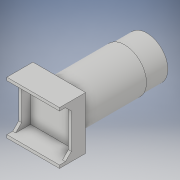
# Autodesk Inventor part: More Accurate Button
Saved by Autodesk Inventor 2018 (Build 220112000, 112)
## iProperties
Created: 2019-09-13
Part Number: More Accurate Button
Material: Generic
Document SubType Name: Modeling
Designer: Jacob
Density: 1 g/cm^3
Appearance: Default
Author: Jacob
Autodesk Inventor part; units mm, degrees
ref_plane "YZ Plane" through (0, 0, 0) normal (1, 0, 0) x (0, 1, 0)
ref_plane "XZ Plane" through (0, 0, 0) normal (0, 1, 0) x (-1, 0, 0)
ref_plane "XY Plane" through (0, 0, 0) normal (0, 0, 1) x (1, 0, 0)
sketch "Sketch1" plane through (0, 0, 0) normal (0, 0, 1) x (1, 0, 0)
  line L0 (-8.875, 8.875) -> (8.875, 8.875)
  line L1 (8.875, 8.875) -> (8.875, -8.875)
  line L2 (8.875, -8.875) -> (-8.875, -8.875)
  line L3 (-8.875, -8.875) -> (-8.875, 8.875)
  line L4 (-8.875, 8.875) -> (8.875, -8.875) construction
  line L5 (8.875, 8.875) -> (-8.875, -8.875) construction
  point P0 (0, 0)
  dimension "d0" = 17.75
  dimension "d1" = 17.75
  constraints: 12 end point, 2 midpoint, 2 parallel, 1 horizontal, 1 perpendicular
  measures "d0" distance of L0.start L0.end
  measures "d1" distance of L0.end L1.end
extrude "Extrusion1" add sketch "Sketch1" along normal blind 8.8
sketch "Sketch2" plane through (0, 0, 0) normal (0, 0, -1) x (-1, 0, 0)
  circle A0 centre (0, 0) radius 7.375
  dimension "d4" = 14.75
  constraints: 1 centre point, 1 coincident
  measures "d4" diameter of A0
extrude "Extrusion2" add sketch "Sketch2" along normal blind 22
sketch "Sketch3" plane through (0, 0, -22) normal (0, 0, -1) x (-1, 0, 0)
  circle A0 centre (0, 0) radius 7.0557
  dimension "d7" = 14.1114
  constraints: 1 centre point, 1 coincident
  measures "d7" diameter of A0
extrude "Extrusion3" add sketch "Sketch3" along normal blind 7.5
sketch "Sketch5" plane through (0, 0, 8.8) normal (0, 0, 1) x (1, 0, 0)
  line L0 (-7.875, 7.875) -> (7.875, 7.875)
  line L1 (7.875, 7.875) -> (7.875, -7.875)
  line L2 (7.875, -7.875) -> (-7.875, -7.875)
  line L3 (-7.875, -7.875) -> (-7.875, 7.875)
  line L4 (-7.875, 7.875) -> (7.875, -7.875) construction
  line L5 (7.875, 7.875) -> (-7.875, -7.875) construction
  line L6 (8.875, 8.875) -> (-8.875, 8.875) projected
  line L7 (8.875, -8.875) -> (8.875, 8.875) projected
  point P0 (0, 0)
  dimension "d14" = 1
  dimension "d15" = 1
  constraints: 12 end point, 2 midpoint, 2 parallel, 1 horizontal, 1 perpendicular
  measures "d14" distance between parallel lines of L6 L0
  measures "d15" distance between parallel lines of L7 L1
extrude "Extrusion5" cut sketch "Sketch5" against normal blind 7
sketch "Sketch6" plane through (0, 0, 8.8) normal (0, 0, 1) x (1, 0, 0)
  line L0 (-7.875, -7.875) -> (-7.875, 7.875) projected
  line L1 (-7.875, 7.875) -> (-8.875, 7.875) construction
  line L2 (-8.875, -8.875) -> (-8.875, 8.875) projected
  line L3 (7.875, 7.875) -> (7.875, -7.875) projected
  line L4 (7.875, 7.875) -> (8.875, 7.875) construction
  line L5 (8.875, -8.875) -> (8.875, 8.875) projected
  line L6 (7.875, -7.875) -> (-7.875, -7.875) projected
  line L7 (-7.875, -7.875) -> (-8.875, -7.875) construction
  line L8 (7.875, -7.875) -> (8.875, -7.875) construction
  line L9 (-8.875, 7.875) -> (8.875, 7.875)
  line L10 (8.875, 7.875) -> (8.875, -7.875)
  line L11 (8.875, -7.875) -> (-8.875, -7.875)
  line L12 (-8.875, -7.875) -> (-8.875, 7.875)
  point P0 (0, 0)
  constraints: 16 end point, 4 point on line, 3 horizontal, 2 parallel, 2 perpendicular
extrude "Extrusion6" cut sketch "Sketch6" against normal blind 4
chamfer "Chamfer1" distance 2 angle 45 4 edges at (8.375, -7.875, 4.8) (-8.375, -7.875, 4.8) (8.375, 7.875, 4.8) (-8.375, 7.875, 4.8)
body "Solid1"
